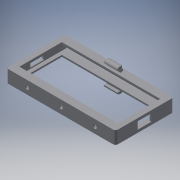
# Autodesk Inventor part: Moto G3 Phone Case version 2
Saved by Autodesk Inventor 2019 (Build 230136000, 136)
## iProperties
Created: 2019-01-09
Part Number: Moto G3 Phone Case version 2
Material: Generic
Document SubType Name: Modeling
Designer: mrhftc
Density: 1 g/cm^3
Appearance: Default
Author: mrhftc
Autodesk Inventor part; units mm, degrees
ref_plane "YZ Plane" through (0, 0, 0) normal (1, 0, 0) x (0, 1, 0)
ref_plane "XZ Plane" through (0, 0, 0) normal (0, 1, 0) x (-1, 0, 0)
ref_plane "XY Plane" through (0, 0, 0) normal (0, 0, 1) x (1, 0, 0)
sketch "Sketch1" plane through (0, 0, 0) normal (0, 1, 0) x (-1, 0, 0)
  line L0 (74.8079, 40.2628) -> (-75.1921, 40.2628)
  line L1 (-75.1921, 40.2628) -> (-75.1921, -39.7372)
  line L2 (-75.1921, -39.7372) -> (74.8079, -39.7372)
  line L3 (74.8079, -39.7372) -> (74.8079, 40.2628)
  line L4 (74.8079, 0.2628) -> (-75.1921, 0.2628) construction
  line L5 (-0.1921, 40.2628) -> (-0.1921, -39.7372) construction
  constraints: 12 end point, 4 midpoint, 2 parallel, 1 horizontal, 1 perpendicular
extrude "Extrusion1" add sketch "Sketch1" along normal blind 17.5
sketch "Sketch2" plane through (0, 17.5, 0) normal (0, 1, 0) x (1, 0, 0)
  line L0 (-67.3032, -29.7573) -> (67.6968, -29.7573)
  line L1 (67.6968, -29.7573) -> (67.6968, 28.6627)
  line L2 (67.6968, 28.6627) -> (-67.3032, 28.6627)
  line L3 (-67.3032, 28.6627) -> (-67.3032, -29.7573)
  line L4 (-74.8079, -40.2628) -> (75.1921, -40.2628) construction
  constraints: 8 end point, 2 parallel, 1 horizontal, 1 perpendicular
extrude "Extrusion2" cut sketch "Sketch2" against normal through all
sketch "Sketch3" plane through (75.1921, 0, -39.7372) normal (0, 0, -1) x (-1, 0, 0)
  line L0 (0, 0) -> (150, 0) construction
  line L1 (147.5, 2.2901) -> (147.5, 14.166)
  line L2 (142.4953, 17.5) -> (142.4953, 0) construction
  line L3 (147.5, 2.2901) -> (2.5, 2.2901)
  line L4 (2.5, 2.2901) -> (2.5, 14.166)
  line L5 (2.5, 14.166) -> (147.5, 14.166)
  point P0 (75.1921, 0)
  point P1 (142.4953, 0.5)
  constraints: 8 end point, 2 perpendicular, 1 parallel
extrude "Extrusion3" cut sketch "Sketch3" against normal blind 77.5
fillet "Fillet1" radius 3.175 4 edges at (-74.8079, 8.75, -39.7372) (75.1921, 8.75, -39.7372) (-74.8079, 8.75, 40.2628) (75.1921, 8.75, 40.2628)
sketch "Sketch4" plane through (0, 17.5, 0) normal (0, 1, 0) x (1, 0, 0)
  line L0 (-9.4891, 36.5622) -> (9.1381, 36.5622)
  line L1 (9.1381, 36.5622) -> (9.1381, 30.374)
  line L2 (9.1381, 30.374) -> (-9.4891, 30.374)
  line L3 (-9.4891, 30.374) -> (-9.4891, 36.5622)
  point P0 (0, 0)
  constraints: 8 end point, 2 parallel, 1 horizontal, 1 perpendicular
extrude "Extrusion4" add sketch "Sketch4" along normal blind 7.62
fillet "Fillet7" radius 3.175 4 edges at (-0.1755, 25.12, -36.5622) (-0.1755, 17.5, -36.5622) (-9.4891, 21.31, -36.5622) (9.1381, 21.31, -36.5622)
sketch "Sketch5" plane through (-9.4891, 17.5, -30.374) normal (0, 0, 1) x (1, 0, 0)
  line L0 (0, 0) -> (0, 7.62) construction
  line L1 (0, 4.3856) -> (18.6272, 4.3856)
  line L2 (18.6272, 4.3856) -> (18.6272, 0)
  line L3 (18.6272, 0) -> (0, 0)
  line L4 (0, 0) -> (0, 4.3856)
  point P0 (9.4891, -17.5)
  constraints: 8 end point, 2 parallel, 1 horizontal, 1 perpendicular, 1 point on line
extrude "Extrusion5" cut sketch "Sketch5" against normal blind 2.032
sketch "Sketch6" plane through (-9.4891, 25.12, -30.374) normal (0, 0, 1) x (1, 0, 0)
  line L0 (0, -3.2344) -> (18.6272, -3.2344)
  line L1 (18.6272, -3.2344) -> (18.6272, 0)
  line L2 (18.6272, 0) -> (0, 0)
  line L3 (0, 0) -> (0, -3.2344)
  point P0 (9.4891, -25.12)
  constraints: 8 end point, 2 parallel, 1 horizontal, 1 perpendicular
extrude "Extrusion6" add sketch "Sketch6" along normal blind 2.032
fillet "Fillet8" radius 3.175 1 edges at (-0.1755, 25.12, -28.342)
sketch "Sketch7" plane through (75.1921, 0, 37.0878) normal (1, 0, 0) x (0, 0, -1)
  line L0 (73.65, 0) -> (73.65, 17.5) construction
  line L1 (65.7506, 0) -> (7.3306, 0) construction
  line L2 (7.3306, 17.5) -> (65.7506, 17.5) construction
  line L3 (46.218, 13.7585) -> (27.432, 13.7585)
  line L4 (27.432, 13.7585) -> (27.432, 3.8084)
  line L5 (27.432, 3.8084) -> (46.218, 3.8084)
  line L6 (46.218, 3.8084) -> (46.218, 13.7585)
  point P0 (37.0878, 0)
  constraints: 8 end point, 2 parallel, 1 horizontal, 1 perpendicular
sketch "Sketch8" plane through (75.1921, 0, 37.7628) normal (0, 0, -1) x (-1, 0, 0)
  line L0 (142.4953, 2.2901) -> (7.4953, 2.2901) construction
  circle A0 centre (121.6243, 8.2281) radius 2.5
  circle A1 centre (28.3826, 8.3252) radius 2.5
  circle A2 centre (75.0026, 8.3682) radius 2.5
  point P0 (75.1921, 0)
  constraints: 3 centre point
extrude "Extrusion8" cut sketch "Sketch8" against normal through all
extrude "Extrusion9" cut sketch "Sketch7" against normal through all
sketch "Sketch11" plane through (0, 0, 0) normal (0, -1, 0) x (1, 0, 0)
  line L0 (9.1381, -28.342) -> (9.1381, -32.406) construction
  line L1 (9.1381, -28.342) -> (-9.4891, -28.342)
  line L2 (-9.4891, -28.342) -> (-9.4891, -36.5622)
  line L3 (-9.4891, -36.5622) -> (9.1381, -36.5622)
  line L4 (9.1381, -36.5622) -> (9.1381, -28.342)
  point P0 (0, 0)
  constraints: 8 end point, 2 parallel, 1 horizontal, 1 perpendicular
extrude "Extrusion12" add sketch "Sketch11" along normal blind 7.62
sketch "Sketch12" plane through (-9.4891, 0, -28.342) normal (0, 0, 1) x (1, 0, 0)
  line L0 (0, 0) -> (0, -7.62) construction
  line L1 (77.186, 0) -> (18.6272, 0) construction
  line L2 (18.6272, 0) -> (0, 0)
  line L3 (0, 0) -> (0, -4.3942)
  line L4 (0, -4.3942) -> (18.6272, -4.3942)
  line L5 (18.6272, -4.3942) -> (18.6272, 0)
  point P0 (9.4891, 0)
  constraints: 8 end point, 2 parallel, 1 horizontal, 1 perpendicular, 1 point on line
extrude "Extrusion13" cut sketch "Sketch12" against normal blind 4.064
fillet "Fillet9" radius 3.175 3 edges at (-0.1755, 0, -36.5622) (-0.1755, -7.62, -36.5622) (-0.1755, -7.62, -28.342)
body "Solid1"
